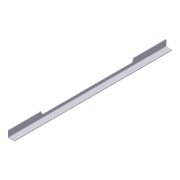
# Autodesk Inventor part: FE-00006-01
Saved by Autodesk Inventor 2012 (Build 160160000, 160)
## iProperties
Created: 2008-05-24
Part Number: FE-00006-01
Document SubType Name: Modeling
Designer: firstuser
Density: 1 g/cm^3
Mass: 1434.14 g
Surface Area: 4677.71 cm^2
Volume: 1434.14 cm^3
Material: Default
Author: firstuser
Autodesk Inventor part; units mm, degrees
ref_plane "YZ Plane" through (0, 0, 0) normal (1, 0, 0) x (0, 1, 0)
ref_plane "XZ Plane" through (0, 0, 0) normal (0, 1, 0) x (-1, 0, 0)
ref_plane "XY Plane" through (0, 0, 0) normal (0, 0, 1) x (1, 0, 0)
sketch "Sketch1" plane through (0, 0, 0) normal (0, 0, 1) x (1, 0, 0)
  line L0 (-25.8536, 31.5645) -> (-25.8536, -44.6355)
  line L1 (-25.8536, -44.6355) -> (50.3464, -44.6355)
  line L2 (50.3464, -44.6355) -> (50.3464, -44.1275)
  line L3 (44.5044, -38.2855) -> (-13.6616, -38.2855)
  line L4 (-19.5036, -32.4435) -> (-19.5036, 25.7225)
  line L5 (-25.3456, 31.5645) -> (-25.8536, 31.5645)
  arc A0 (50.3464, -44.1275) -> (44.5044, -38.2855) centre (44.5044, -44.1275) ccw
  arc A1 (-19.5036, 25.7225) -> (-25.3456, 31.5645) centre (-25.3456, 25.7225) ccw
  arc A2 (-19.5036, -32.4435) -> (-13.6616, -38.2855) centre (-13.6616, -32.4435) ccw
  point P0 (-19.5036, 31.5645)
  dimension "d0" = 76.2
  dimension "d1" = 76.2
  dimension "d2" = 6.35
  dimension "d3" = 5.842
  constraints: 12 end point, 6 point on circle, 6 tangent, 3 centre point, 3 parallel, 2 equal radius, 2 perpendicular, 2 point on line, 1 vertical
  measures "d0" distance of L0.start L0.end
  measures "d1" distance of L0.end L1.end
  measures "d2" distance of point (-19.504, 31.565) L0.start
  measures "d3" radius of A0
extrude "Extrusion1" add sketch "Sketch1" along normal blind 1828.8
sketch "Sketch2" plane through (-25.8536, -44.6355, 0) normal (-1, 0, 0) x (0, 0, 1)
  line L0 (1828.8, 0) -> (1828.8, 76.2) projected
  line L1 (0, 76.2) -> (1828.8, 76.2) projected
  line L2 (0, 76.2) -> (0, 0) projected
  line L3 (0, 0) -> (1828.8, 0) projected
  line L4 (381, 76.2) -> (381, 63.5)
  line L5 (406.4, 38.1) -> (1422.4, 38.1)
  line L6 (1447.8, 63.5) -> (1447.8, 76.2)
  line L7 (1447.8, 76.2) -> (381, 76.2)
  arc A0 (381, 63.5) -> (406.4, 38.1) centre (406.4, 63.5) ccw
  arc A1 (1422.4, 38.1) -> (1447.8, 63.5) centre (1422.4, 63.5) ccw
  dimension "d6" = 25.4
  dimension "d7" = 38.1
  dimension "d8" = 381
  dimension "d9" = 381
  constraints: 8 end point, 4 point on circle, 4 tangent, 2 centre point, 2 parallel, 2 perpendicular, 1 collinear, 1 equal radius
  measures "d6" radius of A0
  measures "d7" distance between parallel lines of L5 L7
  measures "d8" distance between parallel lines of L4 L2
  measures "d9" distance from line of L6.end L0
extrude "Extrusion2" cut sketch "Sketch2" against normal mid plane 1828.8 contours L6 A1 L5 A0 L4 L1
body "Solid1"
